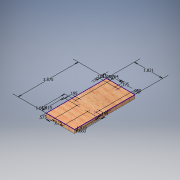
# Autodesk Inventor part: Mousetrap_Base
Saved by Autodesk Inventor 2016 (Build 200138000, 138)
## iProperties
Created: 2017-11-16
Part Number: Mousetrap_Base
Material: Wood (Birch)
Document SubType Name: Modeling
Designer: shen95841
Density: 0.55 g/cm^3
Appearance: Birch - Natural Polished
Author: shen95841
Autodesk Inventor part; units mm, degrees
ref_plane "YZ Plane" through (0, 0, 0) normal (1, 0, 0) x (0, 1, 0)
ref_plane "XZ Plane" through (0, 0, 0) normal (0, 1, 0) x (-1, 0, 0)
ref_plane "XY Plane" through (0, 0, 0) normal (0, 0, 1) x (1, 0, 0)
sketch "Sketch1" plane through (0, 0, 0) normal (0, 1, 0) x (-1, 0, 0)
  line L0 (0, 0) -> (46.2534, 0)
  line L1 (46.2534, 0) -> (46.2534, -98.425)
  line L2 (46.2534, -98.425) -> (0, -98.425)
  line L3 (0, -98.425) -> (0, 0)
  point P0 (31.6992, -36.0426)
  point P1 (14.5542, -36.0426)
  point P2 (39.9034, -42.164)
  point P3 (6.35, -42.164)
  point P4 (39.9034, -47.117)
  point P5 (6.35, -47.117)
  point P6 (26.8478, -92.964)
  point P7 (21.8948, -92.964)
  dimension "d0" = 46.2534
  dimension "d1" = 98.425
  dimension "d2" = 14.5542
  dimension "d3" = 36.0426
  dimension "d4" = 17.145
  dimension "d5" = 36.0426
  dimension "d6" = 6.35
  dimension "d7" = 6.35
  dimension "d8" = 42.164
  dimension "d9" = 42.164
  dimension "d10" = 4.953
  dimension "d11" = 6.35
  dimension "d12" = 6.35
  dimension "d13" = 4.953
  dimension "d14" = 5.461
  dimension "d15" = 19.4056
  dimension "d16" = 4.953
  dimension "d17" = 5.461
  constraints: 8 end point, 2 parallel, 1 horizontal, 1 perpendicular
  measures "d0" distance of L1.end L2.end
  measures "d1" distance of L0.end L1.end
  measures "d2" distance from line of L1 point (31.699, -36.043)
  measures "d3" distance from line of L0 point (31.699, -36.043)
  measures "d4" distance of point (14.554, -36.043) point (31.699, -36.043)
  measures "d5" distance from line of L0 point (14.554, -36.043)
  measures "d6" distance from line of L1 point (39.903, -42.164)
  measures "d7" distance from line of L3 point (6.35, -42.164)
  measures "d8" distance from line of L0 point (39.903, -42.164)
  measures "d9" distance from line of L0 point (6.35, -42.164)
  measures "d10" distance of point (39.903, -42.164) point (39.903, -47.117)
  measures "d11" distance from line of L1 point (39.903, -47.117)
  measures "d12" distance from line of L3 point (6.35, -47.117)
  measures "d13" distance of point (6.35, -42.164) point (6.35, -47.117)
  measures "d14" distance from line of L2 point (26.848, -92.964)
  measures "d15" distance from line of L1 point (26.848, -92.964)
  measures "d16" distance of point (26.848, -92.964) point (21.895, -92.964)
  measures "d17" distance from line of L2 point (21.895, -92.964)
extrude "Extrusion1" add sketch "Sketch1" against normal blind 5.969
hole "Hole1" at (-31.6992, 0, -36.0426) at (-14.5542, 0, -36.0426) at (-39.9034, 0, -42.164) at (-6.35, 0, -42.164) at (-39.9034, 0, -47.117) at (-6.35, 0, -47.117) at (-26.8478, 0, -92.964) at (-21.8948, 0, -92.964) direction (0, -1, 0) diameter 1.397 end through all
body "Solid1"
